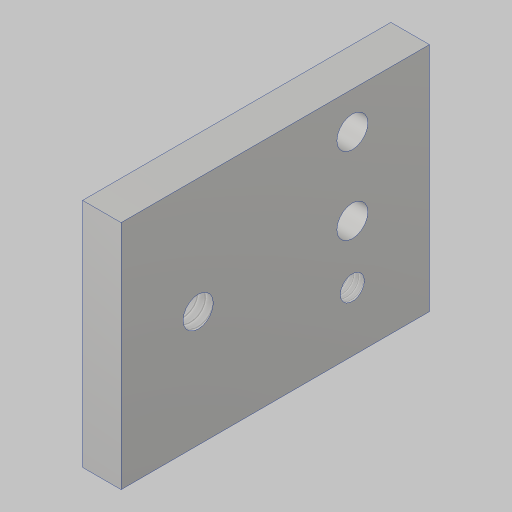
# Autodesk Inventor part: EL2-028
Saved by Autodesk Inventor 2023.5 (Build 275446000, 446)
## iProperties
Created: 2025-02-13
Part Number: EL2-028
Material: Aluminum 6061
Document SubType Name: Modeling
Designer: slick
Density: 2.7 g/cm^3
Appearance: Aluminum - Flat
Author: slick
Autodesk Inventor part; units mm, degrees
ref_plane "YZ Plane" through (0, 0, 0) normal (1, 0, 0) x (0, 1, 0)
ref_plane "XZ Plane" through (0, 0, 0) normal (0, 1, 0) x (-1, 0, 0)
ref_plane "XY Plane" through (0, 0, 0) normal (0, 0, 1) x (1, 0, 0)
sketch "Sketch1" plane through (0, 0, 0) normal (1, 0, 0) x (0, 1, 0)
  line L0 (19.05, 25.4) -> (-19.05, 25.4)
  line L1 (-19.05, 25.4) -> (-19.05, -25.4)
  line L2 (-19.05, -25.4) -> (19.05, -25.4)
  line L3 (19.05, -25.4) -> (19.05, 25.4)
  line L4 (19.05, 25.4) -> (-19.05, -25.4) construction
  line L5 (-19.05, 25.4) -> (19.05, -25.4) construction
  point P0 (0, 0)
  dimension "d0" = 38.1
  dimension "d1" = 50.8
  constraints: 12 end point, 2 midpoint, 2 parallel, 1 horizontal, 1 perpendicular
  measures "d0" distance of L2.end L1.end
  measures "d1" distance of L1.end L0.end
extrude "Extrusion1" add sketch "Sketch1" along normal blind 6.35
sketch "Sketch2" plane through (6.35, 0, 0) normal (1, 0, 0) x (0, 0, -1)
  line L0 (25.4, 19.05) -> (-25.4, 19.05) construction
  line L1 (25.4, -19.05) -> (25.4, 19.05) construction
  point P0 (0, 0)
  point P1 (12.7, 12.954)
  point P2 (12.7, 0.254)
  point P3 (12.7, -9.271)
  dimension "d4" = 12.7
  dimension "d5" = 9.525
  dimension "d6" = 6.096
  dimension "d7" = 12.7
  constraints: 2 vertical alignment
  measures "d4" distance of point (12.7, 0.254) point (12.7, 12.954)
  measures "d5" distance of point (12.7, -9.271) point (12.7, 0.254)
  measures "d6" distance from line of L0 point (12.7, 12.954)
  measures "d7" distance from line of L1 point (12.7, 12.954)
hole "Hole1" at (6.35, 12.954, -12.7) at (6.35, 0.254, -12.7) direction (-1, 0, 0) diameter 5.1054 end through all clearance for "Flat Head Machine Screw (82)" size "#10" standard "Ansi Unified Screw Threads"
hole "Hole2" at (6.35, -9.271, -12.7) direction (-1, 0, 0) diameter 3.9624 end through all thread size "10-32 UNF" class "2B" standard "ANSI Unified Screw Threads"
sketch "Sketch3" plane through (6.35, 0, 0) normal (1, 0, 0) x (0, 0, -1)
  line L0 (-25.4, 19.05) -> (-25.4, -19.05) construction
  point P0 (0, 0)
  point P1 (-12.7, 0)
  dimension "d22" = 12.7
  constraints: 1 horizontal alignment
  measures "d22" distance from line of L0 point (-12.7, 0)
hole "Hole3" at (6.35, 0, 12.7) direction (-1, 0, 0) diameter 4.9784 end through all thread size "1/4-20 UNC" class "2B" standard "ANSI Unified Screw Threads"
body "Solid1"
